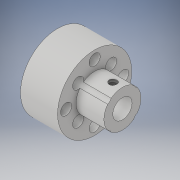
# Autodesk Inventor part: WheelandSprocketComboHub
Saved by Autodesk Inventor 2017 (Build 210142000, 142)
## iProperties
Created: 2018-04-04
Part Number: WheelandSprocketComboHub
Material: Generic
Document SubType Name: Modeling
Designer: User
Density: 1 g/cm^3
Appearance: Default
Author: User
Autodesk Inventor part; units mm, degrees
ref_plane "YZ Plane" through (0, 0, 0) normal (1, 0, 0) x (0, 1, 0)
ref_plane "XY Plane" through (0, 0, 0) normal (0, 0, 1) x (1, 0, 0)
sketch "Sketch1" plane through (0, 0, 0) normal (1, 0, 0) x (0, 1, 0)
  circle A0 centre (0, 0) radius 12.7
  line L0 (5.6576, -5.6576) -> (0, 0)
  line L1 (0, 0.0631) -> (0, -4.7425)
  circle A1 centre (0, 0) radius 3.302
  point P0 (5.6576, 5.6576)
  point P1 (-5.6576, 5.6576)
  point P2 (-5.6576, -5.6576)
  point P3 (9.779, 0)
  point P4 (0, 9.779)
  point P5 (-9.779, 0)
  point P6 (0, -9.779)
  point P7 (5.6576, 5.6576)
  point P8 (-5.6576, 5.6576)
  point P9 (-5.6576, -5.6576)
  dimension "d0" = 25.4
  dimension "d6" = 45
  dimension "d15" = 6.604
  dimension "d23" = 360
  dimension "d25" = 9.779
  dimension "d28" = 360
  constraints: 5 coincident, 4 end point, 2 centre point, 2 point on line, 1 vertical, 10 other
  measures "d0" diameter of A0
  measures "d6" angle of L1 L0
  measures "d15" diameter of A1
  measures "d25" distance of point (0, 0) point (9.779, 0)
extrude "Extrusion1" add sketch "Sketch1" along normal blind 12.7
sketch "Sketch2" plane through (12.7, 0, 0) normal (1, 0, 0) x (0, 0, -1)
  circle A0 centre (0, 0) radius 3.302 projected
  circle A1 centre (0, 0) radius 6.35
  point P0 (0, 0)
  dimension "d18" = 12.7
  constraints: 1 centre point, 1 coincident
  measures "d18" diameter of A1
extrude "Extrusion2" add sketch "Sketch2" along normal blind 9.525
hole "Hole1" at (0, 9.779, 0) at (0, 0, 9.779) at (0, -9.779, 0) at (0, 0, -9.779) direction (1, 0, 0) diameter 3.81 end through all
hole "Hole2" at (0, 5.6576, 5.6576) at (0, -5.6576, 5.6576) at (0, -5.6576, -5.6576) at (0, 5.6576, -5.6576) direction (1, 0, 0) diameter 3.81 end through all
ref_plane "Work Plane2" through (12.7, 6.35, 0) normal (0, 1, 0) x (-1, 0, 0)
sketch "Sketch5" plane through (12.7, 6.35, 0) normal (0, 1, 0) x (-1, 0, 0)
  line L0 (0, 3.8529) -> (-9.525, 3.8529) projected
  line L1 (-9.525, -3.8529) -> (-9.525, 3.8529) projected
  line L2 (-9.525, -3.8529) -> (0, -3.8529) projected
  line L3 (0, 3.8529) -> (0, -3.8529) projected
  point P0 (12.7, 0)
  point P1 (-6.35, 0)
  dimension "d46" = 3.175
  measures "d46" distance from line of point (-6.35, 0) L1
hole "Hole3" at (19.05, 6.35, 0) direction (0, -1, 0) diameter 2.6416 end up to face face through (0, 0, 0) facing (1, 0, 0) round with radius 3.302 far side yes thread size "6-32 UNC" class "2B" standard "ANSI Unified Screw Threads"
body "Solid1"
